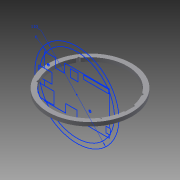
# Autodesk Inventor part: frame
Saved by Autodesk Inventor 2014 (Build 180170000, 170)
## iProperties
Created: 2013-05-24
Part Number: frame
Material: Generisch
Document SubType Name: Modeling
Designer: hartmann
Density: 1 g/cm^3
Appearance: Vorgabe
Author: hartmann
Autodesk Inventor part; units mm, degrees
ref_plane "YZ Plane" through (0, 0, 0) normal (1, 0, 0) x (0, 1, 0)
ref_plane "XZ Plane" through (0, 0, 0) normal (0, 1, 0) x (-1, 0, 0)
ref_plane "XY Plane" through (0, 0, 0) normal (0, 0, 1) x (1, 0, 0)
sketch "Skizze1" plane through (0, 0, 0) normal (0, 0, 1) x (1, 0, 0)
  circle A0 centre (0, 0) radius 49
  circle A1 centre (0, 0) radius 55
  circle A2 centre (-17, -10) radius 1.45 projected
  circle A3 centre (37.5, 15.5) radius 1.45 projected
  line L0 (-37.9, -24) -> (-42.5, -24) projected
  line L1 (-42.5, -24) -> (-42.5, -28) projected
  line L2 (-42.5, -28) -> (-7.5, -28) projected
  line L3 (-7.5, -28) -> (-7.5, -17.2) projected
  line L4 (-7.5, -17.2) -> (7.5, -17.2) projected
  line L5 (7.5, -17.2) -> (7.5, -28) projected
  line L6 (7.5, -28) -> (42.5, -28) projected
  line L7 (42.5, -28) -> (42.5, -26.8) projected
  line L8 (42.5, -26.8) -> (22.5, -26.8) projected
  line L9 (22.5, -26.8) -> (22.5, -10.8) projected
  line L10 (22.5, -10.8) -> (42.5, -10.8) projected
  line L11 (42.5, -10.8) -> (42.5, -4.2) projected
  line L12 (42.5, -4.2) -> (32.6, -4.2) projected
  line L13 (32.6, -4.2) -> (32.6, 9) projected
  line L14 (32.6, 9) -> (42.5, 9) projected
  line L15 (42.5, 9) -> (42.5, 28) projected
  line L16 (42.5, 28) -> (28, 28) projected
  line L17 (28, 28) -> (28, 16.5) projected
  line L18 (28, 16.5) -> (16, 16.5) projected
  line L19 (16, 16.5) -> (16, 28) projected
  line L20 (16, 28) -> (-42.5, 28) projected
  line L21 (-42.5, 28) -> (-42.5, -16.5) projected
  line L22 (-42.5, -16.5) -> (-37.9, -16.5) projected
  line L23 (-37.9, -16.5) -> (-37.9, -24) projected
  line L24 (-8.8, 27) -> (-8.8, 22) projected
  line L25 (-8.8, 22) -> (-41.5, 22) projected
  line L26 (-41.5, 22) -> (-41.5, 27) projected
  line L27 (-41.5, 27) -> (-8.8, 27) projected
  line L28 (-1.5, 15.5) -> (-1.5, 25.5) projected
  line L29 (-1.5, 25.5) -> (8.5, 25.5) projected
  line L30 (8.5, 25.5) -> (8.5, 15.5) projected
  line L31 (8.5, 15.5) -> (-1.5, 15.5) projected
  line L32 (43.5, -10.8) -> (22.5, -10.8) projected
  line L33 (22.5, -10.8) -> (22.5, -26.8) projected
  line L34 (22.5, -26.8) -> (43.5, -26.8) projected
  line L35 (43.5, -26.8) -> (43.5, -10.8) projected
  line L36 (32.6, -4.2) -> (50, -4.2) projected
  line L37 (50, -4.2) -> (50, 9) projected
  line L38 (50, 9) -> (32.6, 9) projected
  line L39 (32.6, 9) -> (32.6, -4.2) projected
  line L40 (-43.5, -24) -> (-37.9, -24) projected
  line L41 (-37.9, -24) -> (-37.9, -16.5) projected
  line L42 (-37.9, -16.5) -> (-43.5, -16.5) projected
  line L43 (-43.5, -16.5) -> (-43.5, -24) projected
  line L44 (43.5, -22.5555) -> (43.5, -26.8)
  line L45 (41.0215, -26.8) -> (43.5, -26.8)
  line L46 (42.5, -26.8) -> (42.5, -28)
  line L47 (40.2119, -28) -> (42.5, -28)
  line L48 (48.8197, -4.2) -> (50, -4.2)
  line L49 (50, -4.2) -> (50, 9)
  line L50 (50, 9) -> (48.1664, 9)
  line L51 (42.5, 24.3875) -> (42.5, 28)
  line L52 (42.5, 28) -> (40.2119, 28)
  line L53 (-42.5, 24.3875) -> (-42.5, 28)
  line L54 (-42.5, 28) -> (-40.2119, 28)
  line L55 (-40.2119, -28) -> (-42.5, -28)
  line L56 (-42.5, -28) -> (-42.5, -24.3875)
  line L57 (-42.72, -24) -> (-43.5, -24)
  line L58 (-43.5, -24) -> (-43.5, -22.5555)
  dimension "d1" = 110
  dimension "d2" = 6
  constraints: 30 end point, 13 point on line, 8 collinear, 2 coincident, 1 centre point, 1 parallel, 1 perpendicular, 15 other
  measures "d1" diameter of A1
extrude "Extrusion3" add sketch "Skizze1" along normal blind 5 contours A1
